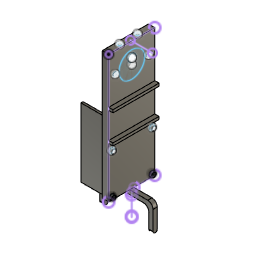
Body (Autodesk Fusion 360 design; units mm, degrees)
Autodesk Fusion 360 part; units mm, degrees
sketch "스케치1" plane through (0, 0, 0) normal (0, 1, 0) x (1, 0, 0)
  line L0 (-25, 0) -> (-25, -25)
  line L1 (-25, -25) -> (25, -25)
  line L2 (25, -25) -> (25, 0)
  line L3 (25, 0) -> (21, 0)
  line L4 (21, 0) -> (21, -21)
  line L5 (21, -21) -> (-21, -21)
  line L6 (-21, -21) -> (-21, 0)
  line L7 (-21, 0) -> (-25, 0)
  constraint vertical L0
  constraint perpendicular L0 L1
  constraint perpendicular L1 L2
  constraint perpendicular L2 L3
  constraint perpendicular L1 L4
  constraint perpendicular L0 L5
  constraint perpendicular L5 L6
  constraint perpendicular L0 L7
extrude "돌출1" add sketch "스케치1" along normal mid plane 4
sketch "스케치2" plane through (0, 0, 25) normal (0, 0, 1) x (-1, 0, 0)
  line L0 (25, 2) -> (-25, 2)
  line L1 (3, -21.65) -> (-3, -21.65)
  line L2 (3, -21.65) -> (3, 0)
  line L3 (-3, -21.65) -> (-3, 0)
  line L4 (-20, 0) -> (-2.5, 0)
  line L5 (3, 21.65) -> (-3, 21.65)
  line L6 (3, 21.65) -> (3, 0)
  line L7 (-3, 21.65) -> (-3, 0)
  line L8 (25, -2) -> (-25, -2)
  dimension "d29" = 21.65
  dimension "d30" = 3
  dimension "d31" = 3
  constraint perpendicular L1 L2
  constraint perpendicular L1 L3
  constraint symmetric L1.start L4 L5.start
  constraint symmetric L1.end L4 L5.end
  constraint symmetric L2.end L4 L6.end
  constraint symmetric L3.end L4 L7.end
  measures "d29" distance of L1 L4
  measures "d30" distance of L2 origin
  measures "d31" distance of origin L3
extrude "돌출2" add sketch "스케치2" along normal blind 120
sketch "스케치14" plane through (0, 0, 145) normal (0, 0, 1) x (-1, 0, 0)
  circle A0 centre (0, -8.4) radius 1.8
  line L0 (-1.75, 0) -> (-22.5, 0)
  circle A1 centre (0, 8.4) radius 1.8
  dimension "d34" = 3.6
  dimension "d35" = 8.4
  constraint symmetric A0 L0 A1
  measures "d34" diameter of A0
  measures "d35" distance of A0.centre L0
extrude "돌출10" cut sketch "스케치14" against normal blind 4.7
thread "스레드1" "ISO Metric profile 3.0 M3x0.5 6H" major diameter 3.086 minor diameter 2.529 pitch 0.5 angle 60 resizes the face on face at (-1.7978, 8.4897, 141.8667)
thread "스레드2" "ISO Metric profile 3.0 M3x0.5 6H" major diameter 3.086 minor diameter 2.529 pitch 0.5 angle 60 resizes the face on face at (-1.7978, -8.3103, 141.8667)
sketch "스케치15" plane through (3, 0, 0) normal (1, 0, 0) x (0, 1, 0)
  line L0 (0, 1.75) -> (0, 22.5)
  line L1 (-21.65, 145) -> (21.65, 145)
  circle A0 centre (-18.85, 27.8) radius 2.25
  line L2 (2, 25) -> (21.65, 25)
  line L3 (-21.65, 25) -> (-21.65, 145)
  circle A1 centre (-18.85, 65.5) radius 2.25
  circle A2 centre (18.85, 65.5) radius 2.25
  circle A3 centre (18.85, 27.8) radius 2.25
  dimension "d43" = 4.5
  dimension "d44" = 2.8
  dimension "d45" = 2.8
  dimension "d46" = 4.5
  dimension "d47" = 37.7
  constraint symmetric L0 A0 A3
  constraint symmetric L0 A1 A2
  measures "d43" diameter of A0
  measures "d44" distance of A0.centre L2
  measures "d45" distance of A0.centre L3
  measures "d46" diameter of A1
  measures "d47" distance of A0.centre A1.centre
extrude "돌출13" add sketch "스케치15" along normal blind 2
sketch "스케치17" plane through (5, 0, 0) normal (1, 0, 0) x (0, 1, 0)
  circle A0 centre (-18.85, 65.5) radius 1.8
  circle A1 centre (-18.85, 27.8) radius 1.8
  line L0 (0, 1.75) -> (0, 22.5)
  circle A2 centre (18.85, 27.8) radius 1.8
  circle A3 centre (18.85, 65.5) radius 1.8
  point P0 (-18.85, 65.5)
  point P1 (-18.85, 27.8)
  dimension "d56" = 3.6
  dimension "d57" = 3.6
  constraint coincident P0 A0.centre
  constraint coincident P1 A1.centre
  constraint symmetric A0 L0 A3
  constraint symmetric A1 L0 A2
  measures "d56" diameter of A0
  measures "d57" diameter of A1
extrude "돌출15" cut sketch "스케치17" against normal blind 4.7
thread "스레드7" "ISO Metric profile 4.0 M4x0.7 6H" major diameter 4.1095 minor diameter 3.332 pitch 0.7 angle 60 resizes the face on face at (1.8667, -17.3141, 66.4386)
thread "스레드8" "ISO Metric profile 4.0 M4x0.7 6H" major diameter 4.1095 minor diameter 3.332 pitch 0.7 angle 60 resizes the face on face at (1.8667, 20.4308, 66.3609)
thread "스레드9" "ISO Metric profile 4.0 M4x0.7 6H" major diameter 4.1095 minor diameter 3.332 pitch 0.7 angle 60 resizes the face on face at (3.4333, -17.0589, 27.6208)
thread "스레드10" "ISO Metric profile 4.0 M4x0.7 6H" major diameter 4.1095 minor diameter 3.332 pitch 0.7 angle 60 resizes the face on face at (1.8667, 20.6478, 27.7103)
sketch "스케치18" plane through (3, 0, 0) normal (1, 0, 0) x (0, 1, 0)
  line L0 (-21.65, 72.3985) -> (21.65, 72.3985)
  line L1 (21.65, 72.3985) -> (21.65, 74.8985)
  line L2 (21.65, 74.8985) -> (-21.65, 74.8985)
  line L3 (-21.65, 74.8985) -> (-21.65, 72.3985)
  line L4 (-21.65, 25) -> (-21.65, 145)
  line L5 (21.65, 25) -> (21.65, 145)
  line L6 (-21.65, 99.3985) -> (21.65, 99.3985)
  line L7 (21.65, 99.3985) -> (21.65, 101.8985)
  line L8 (21.65, 101.8985) -> (-21.65, 101.8985)
  line L9 (-21.65, 101.8985) -> (-21.65, 99.3985)
  dimension "d60" = 2.5
  dimension "d61" = 2.5
  dimension "d62" = 24.5
  constraint horizontal L0
  constraint vertical L1
  constraint horizontal L2
  constraint vertical L3
  constraint coincident L1.end L5
  constraint coincident L0.start L4
  constraint horizontal L6
  constraint vertical L7
  constraint horizontal L8
  constraint vertical L9
  constraint coincident L5 L7.end
  constraint coincident L4 L6.start
  measures "d60" distance of L0.end L1.end
  measures "d61" distance of L6.end L7.end
  measures "d62" distance of L1.end L6.end
extrude "돌출16" add sketch "스케치18" along normal blind 4 contours L0 L1 L2 L3 L4 L5 | L4 L5 L6 L7 L8 L9
sketch "스케치19" plane through (3, 0, 0) normal (1, 0, 0) x (0, 1, 0)
  circle A0 centre (0, 126) radius 12
  circle A1 centre (15.7, 126) radius 1.8
  line L0 (0, 2.5) -> (0, 20)
  circle A2 centre (-15.7, 126) radius 1.8
  circle A3 centre (0, 131.5) radius 3.3
  circle A4 centre (0, 131.5) radius 1.8
  dimension "d65" = 24
  dimension "d66" = 3.6
  dimension "d67" = 15.7
  dimension "d68" = 6.6
  dimension "d69" = 5.5
  dimension "d70" = 3.6
  constraint symmetric A1 L0 A2
  constraint concentric A3 A4
  measures "d65" diameter of A0
  measures "d66" diameter of A1
  measures "d67" distance of A0.centre A1.centre
  measures "d68" diameter of A3
  measures "d69" distance of A0.centre A3.centre
  measures "d70" diameter of A4
extrude "돌출17" cut sketch "스케치19" against normal blind 4.7 contours A1 | A2
extrude "돌출18" cut sketch "스케치19" against normal through all contours A3 | A4
sketch "스케치20" plane through (-3, 0, 0) normal (-1, 0, 0) x (0, -1, 0)
  line L0 (-2, 25) -> (-21.65, 25)
  line L1 (-16.65, 25) -> (-16.65, 89.5)
  line L2 (16.65, 25) -> (16.65, 89.5)
  line L3 (-16.65, 89.5) -> (-18.65, 89.5)
  line L4 (-18.65, 89.5) -> (-18.65, 25)
  line L5 (-18.65, 25) -> (-16.65, 25)
  line L6 (16.65, 25) -> (18.65, 25)
  line L7 (18.65, 25) -> (18.65, 89.5)
  line L8 (18.65, 89.5) -> (16.65, 89.5)
  point P0 (21.65, 25)
  dimension "d74" = 33.3
  dimension "d75" = 5
  dimension "d76" = 5
  dimension "d77" = 2
  dimension "d78" = 2
  dimension "d79" = 64.5
  constraint coincident L0 L1.start
  constraint perpendicular L0 L1
  constraint vertical L2
  constraint perpendicular L1 L3
  constraint coincident L0 L4.end
  constraint perpendicular L0 L4
  constraint perpendicular L2 L6
  constraint perpendicular L6 L7
  constraint perpendicular L2 L8
  measures "d74" distance of L1.end L2.end
  measures "d75" distance of L2.start P0
  measures "d76" distance of L0.end L1.start
  measures "d77" distance of L1.end L3.end
  measures "d78" distance of L2.start L6.end
  measures "d79" distance of L3.end L4.end
extrude "돌출19" add sketch "스케치20" along normal blind 23
fillet "모깎기1" radius 5 4 edges at (-21, 0, 21) (-25, 0, 25) (21, 0, 21) (25, 0, 25)
fillet "모깎기2" radius 2 4 edges at (-23, -2, 0) (-23, 2, 0) (23, -2, 0) (23, 2, 0)
equation "d35 = 10 mm - 1.6 mm"
equation "d67 = 18.5 mm - 2.8 mm"
equation "d69 = 8.5 mm - 3 mm"
